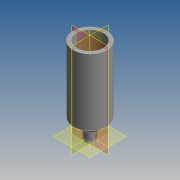
# Autodesk Inventor part: P006_CanonConfettis
Saved by Autodesk Inventor 2020 (Build 240168000, 168)
## iProperties
Created: 2021-10-15
Part Number: P006_CanonConfettis
Material: Générique
Document SubType Name: Modeling
Designer: gabri
Density: 1 g/cm^3
Appearance: Par défaut
Author: gabri
Autodesk Inventor part; units mm, degrees
sketch "Esquisse3" plane through (0, 0, 0) normal (0, 1, 0) x (-1, 0, 0)
  line L0 (-0.25, 6.0789) -> (-0.25, -5.5)
  line L1 (-8, 10) -> (-8, -4)
  line L2 (-8, -4) -> (-5.5, -4)
  line L3 (-5.5, -4) -> (-3, 10)
  line L4 (-3, 10) -> (-8, 10)
  line L5 (0, -31.6) -> (0, 151.1) construction
  line L6 (5.05, 0) -> (-30.3, 0) construction
  line L7 (-3, 10) -> (-20.25, 25)
  line L8 (-20.25, 25) -> (-20.25, 125)
  line L9 (-8, 10) -> (-25.25, 25)
  line L10 (-25.25, 25) -> (-25.25, 125)
  line L11 (-25.25, 125) -> (-20.25, 125)
  line L12 (-30.3, 0) -> (5.05, 0) construction
  point P0 (0, 0)
  dimension "d0" = 5.5
  dimension "d1" = 10.5
  dimension "d2" = 15.5
  dimension "d3" = 14
  dimension "d4" = 8
  dimension "d5" = 10
  dimension "d9" = 40
  dimension "d10" = 15
  dimension "d11" = 100
  dimension "d13" = 5
  dimension "d14" = 5
  dimension "d15" = 125
  constraints: 20 end point, 4 vertical, 2 parallel, 2 perpendicular, 1 other
  measures "d0" diameter of L3.end L0
  measures "d1" diameter of L2.end L0
  measures "d2" diameter of L1 L0
  measures "d3" distance of L1.start L1.end
  measures "d4" distance of the line from the sketch origin of L1
  measures "d5" distance between parallel lines of L6 L4
  measures "d9" diameter of L8 L0
  measures "d10" vertical distance of L3.end L7.end
  measures "d11" distance of L9.end L10.end
  measures "d13" distance between parallel lines of L8 L10
  measures "d14" distance of L3.end L1.start
  measures "d15" distance between parallel lines of L12 L11
revolve "Révolution1" add sketch "Esquisse3" angle 360 about axis through (0.25, 0, 6.0789) along (0, 0, -1)
